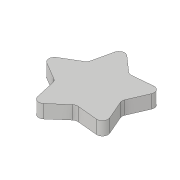
# Autodesk Inventor part: star
Saved by Autodesk Inventor 2019 (Build 230136000, 136)
## iProperties
Created: 2020-06-22
Part Number: star
Material: Generic
Document SubType Name: Modeling
Designer: dmulr
Density: 1 g/cm^3
Appearance: Default
Mass: 19367.9 g
Surface Area: 7981.88 cm^2
Volume: 19367.9 cm^3
Author: dmulr
Autodesk Inventor part; units mm, degrees
ref_plane "YZ Plane" through (0, 0, 0) normal (1, 0, 0) x (0, 1, 0)
ref_plane "XZ Plane" through (0, 0, 0) normal (0, 1, 0) x (-1, 0, 0)
ref_plane "XY Plane" through (0, 0, 0) normal (0, 0, 1) x (1, 0, 0)
sketch "Sketch2" plane through (0, 0, 0) normal (0, 1, 0) x (-1, 0, 0)
  line L0 (450, 0) -> (139.0576, -427.9754) construction
  line L1 (139.0576, -427.9754) -> (-364.0576, -264.5034) construction
  line L2 (-364.0576, -264.5034) -> (-364.0576, 264.5034) construction
  line L3 (-364.0576, 264.5034) -> (139.0576, 427.9754) construction
  line L4 (139.0576, 427.9754) -> (450, 0) construction
  circle A0 centre (0, 0) radius 450 construction
  line L5 (-250, 0) -> (-77.2542, 237.7641) construction
  line L6 (-77.2542, 237.7641) -> (202.2542, 146.9463) construction
  line L7 (202.2542, 146.9463) -> (202.2542, -146.9463) construction
  line L8 (202.2542, -146.9463) -> (-77.2542, -237.7641) construction
  line L9 (-77.2542, -237.7641) -> (-250, 0) construction
  circle A1 centre (0, 0) radius 250 construction
  line L10 (450, 0) -> (202.2542, 146.9463)
  line L11 (139.0576, 427.9754) -> (202.2542, 146.9463)
  line L12 (139.0576, 427.9754) -> (-77.2542, 237.7641)
  line L13 (-77.2542, 237.7641) -> (-364.0576, 264.5034)
  line L14 (-250, 0) -> (-364.0576, 264.5034)
  line L15 (-250, 0) -> (-364.0576, -264.5034)
  line L16 (-77.2542, -237.7641) -> (-364.0576, -264.5034)
  line L17 (202.2542, -146.9463) -> (139.0576, -427.9754)
  line L18 (-77.2542, -237.7641) -> (139.0576, -427.9754)
  line L19 (450, 0) -> (202.2542, -146.9463)
  dimension "d17" = 500
  dimension "d16" = 450
  constraints: 40 end point, 4 coincident, 2 point on circle, 1 centre point, 1 point on line, 25 other
  measures "d16" distance of point (0, 0) L0.start
extrude "Extrusion2" add sketch "Sketch2" along normal mid plane 120
fillet "Fillet1" radius 50 1 edges at (-139.0576, 0, 427.9754)
fillet "Fillet2" radius 50 9 edges at (364.0576, 0, 264.5034) (364.0576, 0, -264.5034) (-139.0576, 0, -427.9754) (-450, 0, 0) (-202.2542, 0, -146.9463) (-202.2542, 0, 146.9463) (77.2542, 0, -237.7641) (250, 0, 0) (77.2542, 0, 237.7641)
body "Solid2"
